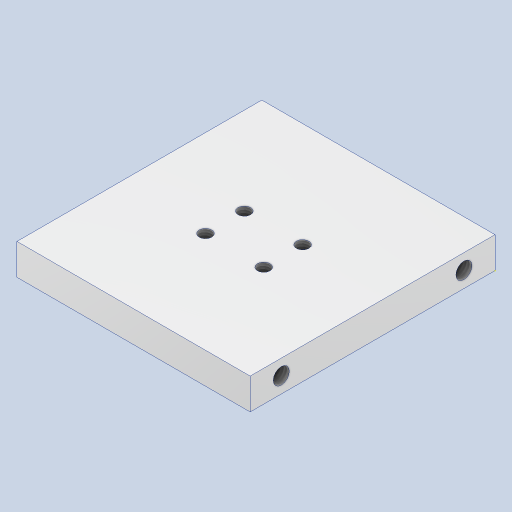
# Autodesk Inventor part: Frente da caixa de susentação
Saved by Autodesk Inventor 2023 (Build 270158000, 158)
## iProperties
Created: 2023-03-23
Part Number: Frente da caixa de susentação
Material: Aluminum 6061
Document SubType Name: Sheet Metal
Designer: 062190003
Density: 2.7 g/cm^3
Sheet Metal Rule: Default_mm
Appearance: Aluminum - Flat
Mass: 78.8163 g
Surface Area: 105.345 cm^2
Volume: 29.1912 cm^3
Author: 062190003
Autodesk Inventor part; units mm, degrees
note: some values were not read from the file. Chosen so that the rebuilt part matches the saved one: direction of "Furo1".
ref_plane "YZ Plane" through (0, 0, 0) normal (1, 0, 0) x (0, 1, 0)
ref_plane "XZ Plane" through (0, 0, 0) normal (0, 1, 0) x (-1, 0, 0)
ref_plane "XY Plane" through (0, 0, 0) normal (0, 0, 1) x (1, 0, 0)
sketch "Sketch1" plane through (0, 0, 0) normal (0, 1, 0) x (-1, 0, 0)
  line L0 (0, 0) -> (60, 0)
  line L1 (60, 0) -> (60, -63)
  line L2 (60, -63) -> (0, -63)
  line L3 (0, -63) -> (0, 0)
  dimension "d0" = 60
  dimension "d1" = 63
  constraints: 8 end point, 2 parallel, 1 horizontal, 1 perpendicular
  measures "d0" distance of L1.end L2.end
  measures "d1" distance of L0.end L1.end
extrude "Extrusion1" add sketch "Sketch1" along normal blind 8
sketch "Esboço2" plane through (0, 8, 0) normal (0, 1, 0) x (1, 0, 0)
  line L0 (0, 63) -> (-60, 63) projected
  line L1 (-60, 63) -> (-60, 0) projected
  line L2 (-60, 0) -> (0, 0) projected
  point P0 (-37.5, 36)
  point P1 (-22.5, 36)
  point P2 (-22.5, 26)
  point P3 (-37.5, 26)
  dimension "d5" = 0
  dimension "d6" = 15
  dimension "d7" = 0
  dimension "d8" = 15
  dimension "d9" = 10
  dimension "d10" = 0
  dimension "d11" = 60
  dimension "d12" = 22.5
  dimension "d20" = 26
  measures "d5" vertical distance of point (-37.5, 36) point (-22.5, 36)
  measures "d6" distance of point (-37.5, 36) point (-22.5, 36)
  measures "d7" horizontal distance of point (-22.5, 26) point (-22.5, 36)
  measures "d8" distance of point (-22.5, 26) point (-37.5, 26)
  measures "d9" distance of point (-37.5, 36) point (-37.5, 26)
  measures "d10" horizontal distance of point (-37.5, 36) point (-37.5, 26)
  measures "d11" distance of L0.start L0.end
  measures "d12" distance from line of L1 point (-37.5, 36)
  measures "d20" distance from line of L2 point (-37.5, 26)
hole "Furo1" at (-37.5, 8, -36) at (-22.5, 8, -36) at (-22.5, 8, -26) at (-37.5, 8, -26) direction (0, -1, 0) diameter 3.242 depth 8 thread size "M4x0.7" class "6H" standard "ISO Metric profile"
sketch "Sketch3" plane through (0, 0, -63) normal (0, 0, -1) x (-1, 0, 0)
  point P0 (0, 0)
sketch "Sketch4" plane through (0, 0, 0) normal (1, 0, 0) x (0, 0, -1)
  line L0 (63, 0) -> (63, 8) projected
  line L1 (0, 0) -> (0, 8) projected
  point P0 (55.0003, 4.0635)
  point P1 (8, 4.0565)
  point P2 (63, 4)
  point P3 (0, 4)
  dimension "d21" = 8
  dimension "d22" = 8
  constraints: 2 midpoint
  measures "d21" distance of point (63, 4) point (55, 4.064)
  measures "d22" horizontal distance of point (0, 4) point (8, 4.056)
hole "Hole2" at (0, 4.0635, -55.0003) at (0, 4.0565, -8) direction (-1, 0, 0) diameter 4.134 depth 14.2 tip angle 118 thread size "M5x0.8" class "6H" standard "ISO Metric profile"
sketch "Sketch5" plane through (-60, 0, -63) normal (-1, 0, 0) x (0, 0, 1)
  circle A0 centre (55, 4.0565) radius 2.067 projected
  circle A1 centre (7.9997, 4.0635) radius 2.067 projected
  point P0 (63, 0)
  constraints: 2 coincident
hole "Hole3" at (-60, 4.0565, -8) at (-60, 4.0635, -55.0003) direction (1, 0, 0) diameter 4.134 depth 14.2 tip angle 118 thread size "M5x0.8" class "6H" standard "ISO Metric profile"
equation "\"d12\" = -0.5 * d6 + 0.5 * d11"
equation "\"d18\" = Thickness"
equation "\"BendRadius\" = Thickness"
equation "\"BendReliefWidth\" = Thickness"
equation "\"BendReliefDepth\" = 0.5 * Thickness"
equation "\"CornerReliefSize\" = 4 * Thickness"
equation "\"MinimumRemnant\" = 2 * Thickness"
equation "\"TransitionRadius\" = BendRadius"
equation "\"JacobiRadiusSize\" = BendRadius"
equation "\"GapSize\" = Thickness"
equation "\"Thickness\" = 0.5"
body "Solid1"
